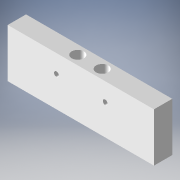
# Autodesk Inventor part: solenoid valve
Saved by Autodesk Inventor 2017 (Build 210142000, 142)
## iProperties
Created: 2016-11-06
Part Number: solenoid valve
Material: PC/ABS Plastic
Document SubType Name: Modeling
Designer: gus
Density: 0.357273 g/cm^3
Appearance: Smooth - White
Author: gus
Autodesk Inventor part; units mm, degrees
ref_plane "YZ Plane" through (0, 0, 0) normal (1, 0, 0) x (0, 1, 0)
ref_plane "XZ Plane" through (0, 0, 0) normal (0, 1, 0) x (-1, 0, 0)
ref_plane "XY Plane" through (0, 0, 0) normal (0, 0, 1) x (1, 0, 0)
sketch "Sketch1" plane through (0, 0, 0) normal (0, 0, 1) x (1, 0, 0)
  line L0 (0, 0) -> (-76.2, 0)
  line L1 (-76.2, 0) -> (-76.2, -25.4)
  line L2 (-76.2, -25.4) -> (0, -25.4)
  line L3 (0, -25.4) -> (0, 0)
  circle A0 centre (-50.8, -9.525) radius 1.27
  circle A1 centre (-25.4, -9.525) radius 1.27
  dimension "d0" = 76.2
  dimension "d1" = 25.4
  dimension "d2" = 25.4
  dimension "d3" = 25.4
  dimension "d4" = 2.54
  dimension "d5" = 9.525
  dimension "d6" = 9.525
  constraints: 8 end point, 2 centre point, 2 parallel, 1 equal radius, 1 horizontal, 1 perpendicular
  measures "d0" distance of L1.end L2.end
  measures "d1" distance of L2.end L0.start
  measures "d2" distance of A1.centre A0.centre
  measures "d3" distance from line of L3 A1.centre
  measures "d4" diameter of A0
  measures "d5" distance from line of L0 A0.centre
  measures "d6" distance from line of L0 A1.centre
extrude "Extrusion1" add sketch "Sketch1" along normal blind 12.7
sketch "Sketch2" plane through (-76.2, 0, 0) normal (0, 1, 0) x (1, 0, 0)
  circle A0 centre (31.75, -6.35) radius 3.175
  circle A1 centre (44.45, -6.35) radius 3.175
  line L0 (0, 0) -> (76.2, 0) projected
  line L1 (0, 0) -> (0, -12.7) projected
  line L2 (76.2, 0) -> (76.2, -12.7) projected
  dimension "d9" = 6.35
  dimension "d10" = 6.35
  dimension "d11" = 6.35
  dimension "d12" = 6.35
  dimension "d13" = 31.75
  dimension "d14" = 31.75
  constraints: 2 centre point
  measures "d9" diameter of A0
  measures "d10" diameter of A1
  measures "d11" distance from line of L0 A0.centre
  measures "d12" distance from line of L0 A1.centre
  measures "d13" distance from line of L1 A0.centre
  measures "d14" distance from line of L2 A1.centre
extrude "Extrusion2" cut sketch "Sketch2" against normal blind 6.35
sketch "Sketch3" plane through (-76.2, -25.4, 0) normal (0, -1, 0) x (1, 0, 0)
  circle A0 centre (38.1, 6.35) radius 3.175
  line L0 (76.2, 0) -> (76.2, 12.7) projected
  line L1 (0, 0) -> (76.2, 0) projected
  dimension "d17" = 6.35
  dimension "d18" = 38.1
  dimension "d19" = 6.35
  constraints: 1 centre point
  measures "d17" diameter of A0
  measures "d18" distance from line of L0 A0.centre
  measures "d19" distance from line of L1 A0.centre
extrude "Extrusion3" cut sketch "Sketch3" against normal blind 6.35
body "Solid1"
